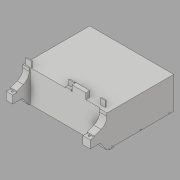
# Autodesk Inventor part: IMA Battery Case Primitive
Saved by Autodesk Inventor 2017 (Build 210142000, 142)
## iProperties
Created: 2021-05-31
Part Number: IMA Battery Case Primitive
Material: Generic
Document SubType Name: Modeling
Designer: Win240
Density: 1 g/cm^3
Appearance: Default
Author: Win240
Autodesk Inventor part; units mm, degrees
ref_plane "YZ Plane" through (0, 0, 0) normal (1, 0, 0) x (0, 1, 0)
ref_plane "XZ Plane" through (0, 0, 0) normal (0, 1, 0) x (-1, 0, 0)
ref_plane "XY Plane" through (0, 0, 0) normal (0, 0, 1) x (1, 0, 0)
sketch "Sketch1" plane through (0, 0, 0) normal (0, 0, 1) x (1, 0, 0)
  line L0 (-212.5, -81.5) -> (212.5, -81.5)
  line L1 (212.5, -81.5) -> (212.5, 81.5)
  line L2 (212.5, 81.5) -> (-212.5, 81.5)
  line L3 (-212.5, 81.5) -> (-212.5, -81.5)
  line L4 (-212.5, -81.5) -> (212.5, 81.5) construction
  line L5 (212.5, -81.5) -> (-212.5, 81.5) construction
  point P0 (0, 0)
  dimension "d0" = 163
  dimension "d1" = 425
  constraints: 12 end point, 2 midpoint, 2 parallel, 1 horizontal, 1 perpendicular
  measures "d0" distance of L0.end L1.end
  measures "d1" distance of L1.end L2.end
extrude "Extrusion1" add sketch "Sketch1" against normal blind 335
sketch "Sketch2" plane through (-212.5, -81.5, 0) normal (0, -1, 0) x (1, 0, 0)
  line L0 (0, 0) -> (425, 0) construction
  line L1 (425, -8) -> (409.5, -8)
  line L2 (409.5, -8) -> (409.5, -28)
  line L3 (409.5, -28) -> (425, -28)
  line L4 (425, -28) -> (425, -8)
  line L5 (20, -10) -> (0, -10)
  line L6 (0, -10) -> (0, -25.5)
  line L7 (0, -25.5) -> (20, -25.5)
  line L8 (20, -25.5) -> (20, -10)
  line L9 (0, -10) -> (0, 0) construction
  line L10 (425, -8) -> (425, 0) construction
  point P0 (212.5, 0)
  dimension "d4" = 8
  dimension "d5" = 10
  dimension "d6" = 15.5
  dimension "d7" = 20
  dimension "d8" = 15.5
  dimension "d9" = 20
  constraints: 20 end point, 4 parallel, 2 horizontal, 2 perpendicular, 2 vertical
  measures "d4" distance between parallel lines of L0 L1
  measures "d5" distance between parallel lines of L5 L0
  measures "d6" distance of L1.start L1.end
  measures "d7" distance of L5.start L5.end
  measures "d8" distance of L7.end L5.start
  measures "d9" distance of L3.end L1.start
extrude "Extrusion2" add sketch "Sketch2" along normal blind 6
sketch "Sketch3" plane through (212.5, -81.5, 0) normal (1, 0, 0) x (0, 0, -1)
  line L0 (0, 0) -> (0, 163) projected
  line L1 (0, 0) -> (-5, 0)
  line L2 (-5, 0) -> (-40, 47)
  line L3 (-40, 47) -> (-90, 47)
  line L4 (-90, 47) -> (-90, 87)
  line L5 (-90, 87) -> (-69, 87)
  line L6 (-69, 93) -> (-34.909, 105.3518)
  line L7 (-69, 87) -> (-69, 93)
  arc A0 (-34.909, 105.3518) -> (-5, 148) centre (-50.3612, 148) ccw
  line L8 (-34.909, 105.3518) -> (0, 118) construction
  arc A1 (-37.8496, 44.1124) -> (-43.6003, 47) centre (-43.6003, 39.8299) ccw
  line L9 (-5, 148) -> (-5, 163)
  line L10 (-5, 163) -> (0, 163)
  dimension "d12" = 5
  dimension "d13" = 47
  dimension "d14" = 35
  dimension "d15" = 40
  dimension "d16" = 90
  dimension "d17" = 118
  dimension "d18" = 93
  dimension "d19" = 69
  dimension "d23" = 55
  dimension "d26" = 5
  dimension "d27" = 15
  constraints: 20 end point, 5 tangent, 4 horizontal, 4 point on circle, 3 point on line, 3 vertical, 2 centre point
  measures "d12" distance of L0.start L1.end
  measures "d13" distance between parallel lines of L1 L3
  measures "d14" horizontal distance of L1.end L2.end
  measures "d15" distance of L3.end L4.end
  measures "d16" distance between parallel lines of L0 L4
  measures "d17" distance from line of L8.end L1
  measures "d18" distance from line of L1 L6.start
  measures "d19" distance between parallel lines of L0 L7
  measures "d23" distance of L1.end A1.start
  measures "d26" distance of L9.end L0.end
  measures "d27" distance of L9.start L9.end
extrude "Extrusion3" add sketch "Sketch3" against normal blind 35
sketch "Sketch4" plane through (-212.5, -81.5, 0) normal (-1, 0, 0) x (0, 0, 1)
  line L0 (0, 0) -> (0, 163) projected
  line L1 (0, 0) -> (5, 0) projected
  line L2 (5, 0) -> (37.8496, 44.1124) projected
  arc A0 (43.6003, 47) -> (37.8496, 44.1124) centre (43.6003, 39.8299) ccw projected
  line L3 (43.6003, 47) -> (90, 47) projected
  line L4 (90, 47) -> (90, 87) projected
  line L5 (90, 87) -> (69, 87) projected
  line L6 (69, 87) -> (69, 93) projected
  line L7 (69, 93) -> (34.909, 105.3518) projected
  arc A1 (5, 148) -> (34.909, 105.3518) centre (50.3612, 148) ccw projected
  line L8 (5, 148) -> (5, 163) projected
  line L9 (5, 163) -> (0, 163) projected
  point P0 (0, 81.5)
extrude "Extrusion4" add sketch "Sketch4" against normal blind 32
sketch "Sketch5" plane through (-212.5, 81.5, -335) normal (0, 1, 0) x (1, 0, 0)
  line L0 (390, -335) -> (32, -335) projected
  line L1 (32, -335) -> (8, -335)
  line L2 (8, -335) -> (8, -330)
  line L3 (8, -330) -> (39, -330)
  line L4 (39, -330) -> (39, -335)
  line L5 (0, 0) -> (0, -340) construction
  point P0 (212.5, -335)
  dimension "d28" = 39
  dimension "d29" = 5
  dimension "d30" = 8
  constraints: 8 end point, 2 horizontal, 2 vertical, 1 point on line
  measures "d28" distance between parallel lines of L4 L5
  measures "d29" distance of L3.end L4.end
  measures "d30" distance between parallel lines of L5 L2
extrude "Extrusion5" add sketch "Sketch5" along normal blind 30
sketch "Sketch6" plane through (-212.5, 81.5, -335) normal (0, 1, 0) x (1, 0, 0)
  line L0 (0, 0) -> (0, -340) construction
  line L1 (390, -335) -> (39, -335) projected
  line L2 (212, -335) -> (212, -315)
  line L3 (212, -315) -> (240, -315)
  line L4 (240, -315) -> (240, -335)
  point P0 (212.5, -335)
  dimension "d33" = 212
  dimension "d34" = 240
  dimension "d35" = 20
  constraints: 6 end point, 2 point on line, 2 vertical, 1 horizontal
  measures "d33" distance between parallel lines of L0 L2
  measures "d34" distance between parallel lines of L4 L0
  measures "d35" distance between parallel lines of L1 L3
extrude "Extrusion6" add sketch "Sketch6" along normal blind 5
sketch "Sketch7" plane through (0, 0, 0) normal (0, 0, 1) x (1, 0, 0)
  line L0 (177.5, 81.5) -> (27.5, 81.5) projected
  line L1 (32.5, 81.5) -> (32.5, 111.5)
  line L2 (-212.5, -81.5) -> (-212.5, 81.5) construction
  line L3 (102.5, 81.5) -> (102.5, 111.5)
  line L4 (32.5, 111.5) -> (102.5, 111.5)
  point P0 (0, 0)
  dimension "d38" = 245
  dimension "d39" = 315
  dimension "d40" = 30
  constraints: 6 end point, 2 vertical, 1 horizontal, 1 midpoint, 1 point on line
  measures "d38" distance from line of L1.start L2
  measures "d39" distance from line of L3.start L2
  measures "d40" distance of L3.start L3.end
extrude "Extrusion7" add sketch "Sketch7" against normal blind 20
sketch "Sketch8" plane through (-212.5, 81.5, -335) normal (0, 1, 0) x (1, 0, 0)
  line L0 (0, 0) -> (0, -340) construction
  line L1 (374, -315) -> (399, -315)
  line L2 (399, -315) -> (399, -320)
  line L3 (399, -320) -> (374, -320)
  line L4 (374, -320) -> (374, -315)
  line L5 (390, -335) -> (315, -335) construction
  point P0 (212.5, -335)
  dimension "d43" = 374
  dimension "d44" = 399
  dimension "d45" = 15
  dimension "d46" = 20
  constraints: 8 end point, 2 parallel, 1 horizontal, 1 perpendicular
  measures "d43" distance between parallel lines of L0 L4
  measures "d44" distance between parallel lines of L2 L0
  measures "d45" distance between parallel lines of L3 L5
  measures "d46" distance between parallel lines of L1 L5
extrude "Extrusion8" add sketch "Sketch8" along normal blind 30
sketch "Sketch9" plane through (-212.5, 86.5, -335) normal (0, 1, 0) x (1, 0, 0)
  line L0 (240, -315) -> (212, -315) projected
  line L1 (240, -335) -> (240, -315) projected
  line L2 (212, -320) -> (240, -320)
  line L3 (212, -315) -> (212, -320)
  line L4 (8, -330) -> (8, -335) construction
  point P0 (212.5, -335)
  constraints: 4 end point, 1 horizontal, 1 parallel, 1 point on line, 1 vertical
extrude "Extrusion9" add sketch "Sketch9" along normal up to surface (25 mm away)
sketch "Sketch10" plane through (-212.5, 5.5, 90) normal (0, 1, 0) x (1, 0, 0)
  line L0 (0, 0) -> (32, 0) projected
  line L1 (425, 0) -> (390, 0) projected
  circle A0 centre (16, 14) radius 4
  circle A1 centre (407.5, 14) radius 4
  line L2 (390, 0) -> (407.5, 14) construction
  line L3 (407.5, 14) -> (425, 0) construction
  line L4 (32, 0) -> (16, 14) construction
  line L5 (16, 14) -> (0, 0) construction
  line L6 (16, 14) -> (407.5, 14) construction
  point P0 (212.5, 90)
  dimension "d51" = 8
  dimension "d52" = 14
  constraints: 10 end point, 2 centre point, 2 equal length, 1 equal radius, 1 horizontal
  measures "d51" diameter of A1
  measures "d52" distance between parallel lines of L6 L0
extrude "Extrusion10" cut sketch "Sketch10" against normal up to surface (40 mm away)
sketch "Sketch11" plane through (212.5, -81.5, -335) normal (1, 0, 0) x (0, 0, -1)
  line L0 (-327, -6) -> (-327, 0) projected
  line L1 (-327, 0) -> (-340, 0) projected
  line L2 (-340, 0) -> (-372.8496, 44.1124) projected
  arc A0 (-372.8496, 44.1124) -> (-378.6003, 47) centre (-378.6003, 39.8299) ccw projected
  line L3 (-378.6003, 47) -> (-425, 47) projected
  line L4 (-425, 47) -> (-425, 87) projected
  line L5 (-425, 87) -> (-404, 87) projected
  line L6 (-404, 87) -> (-404, 93) projected
  line L7 (-404, 93) -> (-369.909, 105.3518) projected
  arc A1 (-369.909, 105.3518) -> (-340, 148) centre (-385.3612, 148) ccw projected
  line L8 (-340, 148) -> (-340, 163) projected
  line L9 (-340, 163) -> (0, 163) projected
  line L10 (0, 163) -> (0, 0) projected
  line L11 (0, 0) -> (-307, 0) projected
  line L12 (-307, 0) -> (-307, -6) projected
  line L13 (-307, -6) -> (-327, -6) projected
  point P0 (-335, 81.5)
extrude "Extrusion11" add sketch "Sketch11" along normal blind 2.5
sketch "Sketch12" plane through (215, -81.5, -335) normal (1, 0, 0) x (0, 0, -1)
  line L0 (-415, 87) -> (-407, 87) construction
  line L1 (-411, 87) -> (-411, 3) construction
  line L2 (-411, 3) -> (-316, 3) construction
  line L3 (-316, 3) -> (-169, 3) construction
  line L4 (-169, 3) -> (-22, 3) construction
  circle A0 centre (-316, 3) radius 3
  circle A1 centre (-169, 3) radius 3
  circle A2 centre (-22, 3) radius 3
  line L5 (-327, -6) -> (-307, -6) projected
  point P0 (-335, 81.5)
  dimension "d57" = 95
  dimension "d58" = 242
  dimension "d59" = 389
  dimension "d60" = 6
  dimension "d63" = 9
  constraints: 8 end point, 3 centre point, 3 coincident, 2 equal radius, 2 horizontal, 1 midpoint, 1 point on line, 1 vertical
  measures "d57" distance of L1.end L2.end
  measures "d58" distance from line of L1 L3.end
  measures "d59" distance from line of L1 L4.end
  measures "d60" diameter of A0
  measures "d63" distance between parallel lines of L2 L5
extrude "Extrusion12" cut sketch "Sketch12" against normal blind 10
body "Solid1"
